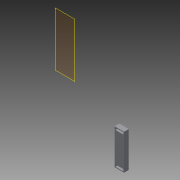
# Autodesk Inventor part: side piece
Saved by Autodesk Inventor 2015 (Build 190159000, 159)
## iProperties
Created: 2014-11-22
Part Number: side piece
Material: Generic
Document SubType Name: Modeling
Designer: jesse
Density: 1 g/cm^3
Appearance: Default
Author: jesse
Autodesk Inventor part; units mm, degrees
ref_plane "YZ Plane" through (0, 0, 0) normal (1, 0, 0) x (0, 1, 0)
ref_plane "XZ Plane" through (0, 0, 0) normal (0, 1, 0) x (-1, 0, 0)
ref_plane "XY Plane" through (0, 0, 0) normal (0, 0, 1) x (1, 0, 0)
ref_plane "Work Plane1" through (29.6407, 50.9726, 24.365) normal (0, 0, -1) x (-1, 0, 0)
sketch "Sketch1" plane through (29.6407, 50.9726, 24.365) normal (0, 0, -1) x (-1, 0, 0)
  line L0 (12.7, 3.175) -> (-12.7, 3.175) projected
  line L1 (-12.7, 3.175) -> (-12.7, -3.175) projected
  line L2 (-12.7, -3.175) -> (12.7, -3.175) projected
  line L3 (12.7, -3.175) -> (12.7, 3.175) projected
  line L4 (-12.7, -113.4117) -> (12.7, -113.4117) projected
  line L5 (12.7, -113.4117) -> (12.7, -107.0617) projected
  line L6 (12.7, -107.0617) -> (-12.7, -107.0617) projected
  line L7 (-12.7, -107.0617) -> (-12.7, -113.4117) projected
  line L8 (-15.24, -5.715) -> (-15.24, 5.715)
  line L9 (-15.24, 5.715) -> (15.24, 5.715)
  line L10 (15.24, 5.715) -> (15.24, -5.715)
  line L11 (15.24, -96.743) -> (15.24, -115.9518)
  line L12 (15.24, -115.9518) -> (-15.24, -115.9518)
  line L13 (-15.24, -115.9518) -> (-15.24, -96.743)
  line L14 (-15.24, -5.715) -> (-15.24, -96.743)
  line L15 (15.24, -5.715) -> (15.24, -98.1393)
  point P0 (29.6407, -50.9726)
  constraints: 16 end point, 1 point on line, 4 other
extrude "Extrusion1" add sketch "Sketch1" against normal blind 12.7
sketch "Sketch2" plane through (29.6407, 50.9726, 24.365) normal (0, 0, -1) x (-1, 0, 0)
  line L0 (15.24, -115.9518) -> (15.24, 5.715) projected
  line L1 (-15.24, -115.9518) -> (15.24, -115.9518) projected
  line L2 (-15.24, 5.715) -> (-15.24, -115.9518) projected
  line L3 (15.24, 5.715) -> (-15.24, 5.715) projected
  point P0 (29.6407, -50.9726)
extrude "Extrusion2" add sketch "Sketch2" along normal blind 2.54
body "Solid1"
